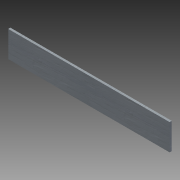
# Autodesk Inventor part: Front
Saved by Autodesk Inventor 2011 SP1 (Build 150282100, 282)
## iProperties
Created: 2011-05-30
Part Number: Front
Document SubType Name: Modeling
Designer: Andrew G. Meyer
Mass: 28.4213 g
Surface Area: 196.371 cm^2
Volume: 28.4213 cm^3
Density: 1 g/cm^3
Author: Andrew G. Meyer
Autodesk Inventor part; units mm, degrees
ref_plane "YZ Plane" through (0, 0, 0) normal (1, 0, 0) x (0, 1, 0)
ref_plane "XZ Plane" through (0, 0, 0) normal (0, 1, 0) x (-1, 0, 0)
ref_plane "XY Plane" through (0, 0, 0) normal (0, 0, 1) x (1, 0, 0)
sketch "Sketch1" plane through (0, 0, 0) normal (0, 0, 1) x (1, 0, 0)
  line L0 (-117.475, 19.05) -> (117.475, 19.05)
  line L1 (117.475, 19.05) -> (117.475, -19.05)
  line L2 (117.475, -19.05) -> (-117.475, -19.05)
  line L3 (-117.475, -19.05) -> (-117.475, 19.05)
  point P0 (0, 0)
  dimension "d0" = 234.95
  dimension "d1" = 117.475
  dimension "d2" = 38.1
  dimension "d3" = 19.05
  constraints: 8 end point, 2 parallel, 1 horizontal, 1 perpendicular
  measures "d0" distance of L0.start L0.end
  measures "d1" distance from line of L3 point (0, 0)
  measures "d2" distance of L2.end L0.start
  measures "d3" distance from line of L0 point (0, 0)
extrude "Extrusion1" add sketch "Sketch1" against normal blind 3.175
equation "\"d1\" = 0.5 * d0"
equation "\"d3\" = 0.5 * d2"
body "Solid1"
